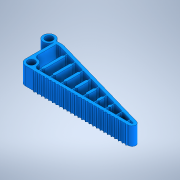
# Autodesk Inventor part: BRAÇO ROBÓTICO - Garra A2
Saved by Autodesk Inventor 2021 (Build 250183000, 183)
## iProperties
Created: 2020-08-23
Part Number: BRAÇO ROBÓTICO - Garra A2
Material: Borracha
Document SubType Name: Modeling
Designer: Araújo, I.
Mass: 6.12763 g
Surface Area: 83.3461 cm^2
Volume: 6.58885 cm^3
Density: 0.93 g/cm^3
Appearance: Borracha - Preta
Author: Araújo, I.
## iProperties of the stored document _3DPrint.ipt
Created: 2020-11-23
Part Number: _3DPrint
Material: Genérico
Document SubType Name: Modeling
Designer: Araújo, I.
Mass: 6.58885 g
Surface Area: 83.3461 cm^2
Volume: 6.58885 cm^3
Density: 1 g/cm^3
Appearance: Padrão
Author: Araújo, I.
Autodesk Inventor part; units mm, degrees
ref_plane "YZ Plane" through (0, 0, 0) normal (1, 0, 0) x (0, 1, 0)
ref_plane "XZ Plane" through (0, 0, 0) normal (0, 1, 0) x (-1, 0, 0)
ref_plane "XY Plane" through (0, 0, 0) normal (0, 0, 1) x (1, 0, 0)
sketch "Esboço1" plane through (0, 0, 0) normal (0, 1, 0) x (-1, 0, 0)
  line L0 (-70.6891, -3.9032) -> (-1.5487, -23.7288)
  arc A0 (-70, 1) -> (-70.6891, -3.9032) centre (-70, -1.5) ccw
  line L1 (-0.9975, -21.8063) -> (-70.1378, -1.9806)
  line L2 (-70, -1) -> (-6, -1)
  line L3 (-7, -20.0851) -> (-7, -18.0851)
  line L4 (-7, -18.0851) -> (-6.4, -17.4851)
  line L5 (-6.4, -17.4851) -> (-6.4, -3.6)
  line L6 (-6.4, -3.6) -> (-7, -3)
  line L7 (-7, -3) -> (-7, -1)
  line L8 (-7.8, -1) -> (-7.8, -3)
  line L9 (-7.8, -3) -> (-8.4, -3.6)
  line L10 (-8.4, -3.6) -> (-8.4, -17.4851)
  line L11 (-8.4, -17.4851) -> (-7.8, -18.0851)
  line L12 (-7.8, -18.0851) -> (-7.8, -19.8557)
  line L13 (-14.5, -17.9345) -> (-14.5, -15.9345)
  line L14 (-14.5, -15.9345) -> (-13.9, -15.3345)
  line L15 (-13.9, -15.3345) -> (-13.9, -3.6)
  line L16 (-13.9, -3.6) -> (-14.5, -3)
  line L17 (-14.5, -3) -> (-14.5, -1)
  line L18 (-15.3, -1) -> (-15.3, -3)
  line L19 (-15.3, -3) -> (-15.9, -3.6)
  line L20 (-15.9, -3.6) -> (-15.9, -15.3345)
  line L21 (-15.9, -15.3345) -> (-15.3, -15.9345)
  line L22 (-15.3, -15.9345) -> (-15.3, -17.7051)
  line L23 (-21.4, -13.1839) -> (-21.4, -3.6)
  line L24 (-23.4, -3.6) -> (-23.4, -13.1839)
  line L25 (-21.4, -3.6) -> (-22, -3)
  line L26 (-22.8, -3) -> (-23.4, -3.6)
  line L27 (-22, -3) -> (-22, -1)
  line L28 (-22.8, -1) -> (-22.8, -3)
  line L29 (-22.8, -13.7839) -> (-22.8, -15.5545)
  line L30 (-23.4, -13.1839) -> (-22.8, -13.7839)
  line L31 (-22, -15.7839) -> (-22, -13.7839)
  line L32 (-22, -13.7839) -> (-21.4, -13.1839)
  line L33 (-28.9, -11.0333) -> (-28.9, -3.6)
  line L34 (-30.9, -3.6) -> (-30.9, -11.0333)
  line L35 (-28.9, -3.6) -> (-29.5, -3)
  line L36 (-30.3, -3) -> (-30.9, -3.6)
  line L37 (-29.5, -3) -> (-29.5, -1)
  line L38 (-30.3, -1) -> (-30.3, -3)
  line L39 (-30.3, -11.6333) -> (-30.3, -13.4039)
  line L40 (-30.9, -11.0333) -> (-30.3, -11.6333)
  line L41 (-29.5, -13.6333) -> (-29.5, -11.6333)
  line L42 (-29.5, -11.6333) -> (-28.9, -11.0333)
  line L43 (-36.4, -8.8827) -> (-36.4, -3.6)
  line L44 (-38.4, -3.6) -> (-38.4, -8.8827)
  line L45 (-36.4, -3.6) -> (-37, -3)
  line L46 (-37.8, -3) -> (-38.4, -3.6)
  line L47 (-37, -3) -> (-37, -1)
  line L48 (-37.8, -1) -> (-37.8, -3)
  line L49 (-37.8, -9.4827) -> (-37.8, -11.2534)
  line L50 (-38.4, -8.8827) -> (-37.8, -9.4827)
  line L51 (-37, -11.4827) -> (-37, -9.4827)
  line L52 (-37, -9.4827) -> (-36.4, -8.8827)
  line L53 (-43.9, -6.7322) -> (-43.9, -3.6)
  line L54 (-45.9, -3.6) -> (-45.9, -6.7322)
  line L55 (-43.9, -3.6) -> (-44.5, -3)
  line L56 (-45.3, -3) -> (-45.9, -3.6)
  line L57 (-44.5, -3) -> (-44.5, -1)
  line L58 (-45.3, -1) -> (-45.3, -3)
  line L59 (-45.3, -7.3322) -> (-45.3, -9.1028)
  line L60 (-45.9, -6.7322) -> (-45.3, -7.3322)
  line L61 (-44.5, -9.3322) -> (-44.5, -7.3322)
  line L62 (-44.5, -7.3322) -> (-43.9, -6.7322)
  line L63 (-51.4, -4.5816) -> (-51.4, -3.6)
  line L64 (-53.4, -3.6) -> (-53.4, -4.5816)
  line L65 (-52, -5.1816) -> (-51.4, -4.5816)
  line L66 (-53.4, -4.5816) -> (-52.8, -5.1816)
  line L67 (-52, -7.1816) -> (-52, -5.1816)
  line L68 (-52.8, -5.1816) -> (-52.8, -6.9522)
  line L69 (-52.8, -3) -> (-53.4, -3.6)
  line L70 (-51.4, -3.6) -> (-52, -3)
  line L71 (-52.8, -1) -> (-52.8, -3)
  line L72 (-52, -3) -> (-52, -1)
  arc A1 (-70, -1) -> (-70.1378, -1.9806) centre (-70, -1.5) ccw
  line L73 (-59.5, -3) -> (-59.5, -1)
  line L74 (-60.3, -1) -> (-60.3, -3)
  line L75 (-58.9, -3.6) -> (-59.5, -3)
  line L76 (-58.9, -2.431) -> (-58.9, -3.6)
  line L77 (-60.3, -3) -> (-60.9, -3.6)
  line L78 (-60.9, -3.6) -> (-60.9, -2.431)
  line L79 (-59.5, -3.031) -> (-58.9, -2.431)
  line L80 (-60.9, -2.431) -> (-60.3, -3.031)
  line L81 (-59.5, -5.031) -> (-59.5, -3.031)
  line L82 (-60.3, -3.031) -> (-60.3, -4.8016)
  line L83 (-67, -2.8804) -> (-67, -1)
  line L84 (-67.8, -2.651) -> (-67.8, -1)
  line L85 (-74.5, -0.7298) -> (-74.5, -1)
  line L86 (-75.3, -0.5004) -> (-75.3, -1)
  circle A2 centre (8, -23) radius 2.5
  arc A3 (4.127, -24) -> (4.127, -22) centre (8, -23) ccw
  line L87 (4.127, -24) -> (0.3807, -24)
  line L88 (4.127, -24) -> (4.127, -22) construction
  arc A4 (-0.9975, -21.8063) -> (0.3807, -22) centre (0.3807, -17) ccw
  arc A5 (-1.5487, -23.7288) -> (0.3807, -24) centre (0.3807, -17) ccw
  circle A6 centre (0, -3) radius 2.5
  line L89 (0, 1) -> (-70, 1)
  arc A7 (-4, -3) -> (-6, -1) centre (-6, -3) ccw
  line L90 (4, -3) -> (4, -22)
  line L91 (2, -9) -> (2, -22)
  arc A8 (-4, -3) -> (0, -7) centre (0, -3) ccw
  arc A9 (4, -3) -> (0, 1) centre (0, -3) ccw
  arc A10 (2, -9) -> (0, -7) centre (0, -9) ccw
  line L92 (4.127, -22) -> (4, -22)
  line L93 (2, -22) -> (0.3807, -22)
  line L94 (-6, -1) -> (-6, 1) construction
  point P0 (4.127, -23)
  point P1 (0, 0)
  point P2 (-6, 0)
  point P3 (-60.3155, -3.0155)
  point P4 (-59.4845, -3.0155)
  dimension "d194" = 16
  dimension "d4" = 2.5
  dimension "d6" = 2
  dimension "d39" = 0.8
  dimension "d40" = 2
  dimension "d41" = 2
  dimension "d44" = 45
  dimension "d46" = 0.8
  dimension "d47" = 2
  dimension "d48" = 2
  dimension "d49" = 45
  dimension "d53" = 7.5
  dimension "d54" = 0.8
  dimension "d55" = 2
  dimension "d56" = 2
  dimension "d57" = 45
  dimension "d63" = 0.8
  dimension "d64" = 2
  dimension "d65" = 2
  dimension "d66" = 45
  dimension "d72" = 0.8
  dimension "d73" = 2
  dimension "d74" = 2
  dimension "d75" = 45
  dimension "d81" = 0.8
  dimension "d82" = 2
  dimension "d83" = 2
  dimension "d84" = 45
  dimension "d117" = 7.5
  dimension "d119" = 7.5
  dimension "d120" = 7.5
  dimension "d124" = 7.5
  dimension "d125" = 0.8
  dimension "d126" = 2
  dimension "d127" = 2
  dimension "d128" = 45
  dimension "d155" = 7.5
  dimension "d157" = 0.8
  dimension "d158" = 2
  dimension "d159" = 2
  dimension "d160" = 45
  dimension "d167" = 7.5
  dimension "d168" = 0.8
  dimension "d169" = 0.8
  dimension "d170" = 7.5
  dimension "d171" = 7.5
  dimension "d183" = 5
  dimension "d184" = 1.5
  dimension "d189" = 5
  dimension "d220" = 5
  dimension "d222" = 70
  dimension "d223" = 20
  dimension "d224" = 8
  dimension "d225" = 7
  dimension "d227" = 2
  dimension "d235" = 2
  dimension "d237" = 1.5
  constraints: 186 end point, 33 point on line, 32 equal length, 21 vertical, 18 horizontal alignment, 18 point on circle, 16 parallel, 13 perpendicular, 11 centre point, 11 tangent, 4 horizontal, 3 coincident, 2 equal radius, 2 midpoint, 1 concentric, 1 vertical alignment, 50 other
  measures "d4" radius of A0
  measures "d39" distance between parallel lines of L8 L7
  measures "d40" distance between parallel lines of L10 L5
  measures "d41" distance of L6.end L7.end
  measures "d44" angle of L11 L12
  measures "d46" distance between parallel lines of L18 L17
  measures "d47" distance between parallel lines of L20 L15
  measures "d48" distance of L16.end L17.end
  measures "d49" angle of L21 L22
  measures "d53" distance between parallel lines of L13 L3
  measures "d54" distance between parallel lines of L28 L27
  measures "d55" distance between parallel lines of L24 L23
  measures "d56" distance of L25.end L27.end
  measures "d57" angle of L30 L29
  measures "d63" distance between parallel lines of L38 L37
  measures "d64" distance between parallel lines of L34 L33
  measures "d65" distance of L35.end L37.end
  measures "d66" angle of L40 L39
  measures "d72" distance between parallel lines of L48 L47
  measures "d73" distance between parallel lines of L44 L43
  measures "d74" distance of L45.end L47.end
  measures "d75" angle of L50 L49
  measures "d81" distance between parallel lines of L58 L57
  measures "d82" distance between parallel lines of L54 L53
  measures "d83" distance of L55.end L57.end
  measures "d84" angle of L60 L59
  measures "d117" distance between parallel lines of L31 L13
  measures "d119" distance between parallel lines of L41 L31
  measures "d120" distance between parallel lines of L51 L41
  measures "d124" distance between parallel lines of L61 L51
  measures "d125" distance between parallel lines of L71 L72
  measures "d126" distance between parallel lines of L64 L63
  measures "d127" distance of L72.start L72.end
  measures "d128" angle of L66 L68
  measures "d155" distance between parallel lines of L67 L61
  measures "d157" distance between parallel lines of L74 L73
  measures "d158" distance between parallel lines of L78 L76
  measures "d159" distance of L73.start L73.end
  measures "d160" angle of L80 L82
  measures "d167" distance between parallel lines of L81 L67
  measures "d168" distance between parallel lines of L84 L83
  measures "d169" distance between parallel lines of L86 L85
  measures "d170" distance between parallel lines of L83 L81
  measures "d171" distance between parallel lines of L85 L83
  measures "d183" diameter of A2
  measures "d184" radial gap between concentric circles of A2 A3
  measures "d189" radius of A4
  measures "d220" diameter of A6
  measures "d222" horizontal distance of A1.centre point (0, 0)
  measures "d223" vertical distance of A6.centre A2.centre
  measures "d224" horizontal distance of A6.centre A2.centre
  measures "d225" distance from line of L3 A6.centre
  measures "d227" radius of A7
  measures "d235" distance between parallel lines of L91 L90
  measures "d237" radial gap between concentric circles of A8 A6
extrude "Extrusão1" add sketch "Esboço1" along normal blind 12 contours A0 L89 A9 L90 L92 A3 L87 A5 L0 | L1 L12 L11 L10 L9 L8 L2 L7 L6 L5 L4 L3 | L1 L22 L21 L20 L19 L18 L2 L17 L16 L15 L14 L13 | L1 L29 L30 L24 L26 L28 L2 L27 L25 L23 L32 L31 | L1 L39 L40 L34 L36 L38 L2 L37 L35 L33 L42 L41 | L1 L49 L50 L44 L46 L48 L2 L47 L45 L43 L52 L51 | L1 L59 L60 L54 L56 L58 L2 L57 L55 L53 L62 L61 | L1 L68 L66 L64 L69 L71 L2 L72 L70 L63 L65 L67 | L1 L82 L80 L77 L74 L2 L73 L75 L79 L81 | L1 L84 L2 L83
sketch "Esboço2" plane through (0, 0, 0) normal (0, 1, 0) x (-1, 0, 0)
  line L0 (-5.8804, 1) -> (-6.3134, 1.75)
  line L1 (-6.4866, 1.75) -> (-6.9196, 1)
  line L2 (-6.9196, 1) -> (-5.8804, 1)
  arc A0 (-6.3134, 1.75) -> (-6.4866, 1.75) centre (-6.4, 1.7) ccw
  line L3 (0, 1) -> (-70, 1) projected
  line L4 (-8.3804, 1) -> (-8.8134, 1.75)
  arc A1 (-8.8134, 1.75) -> (-8.9866, 1.75) centre (-8.9, 1.7) ccw
  line L5 (-8.9866, 1.75) -> (-9.4196, 1)
  line L6 (-9.4196, 1) -> (-8.3804, 1)
  line L7 (-10.8804, 1) -> (-11.3134, 1.75)
  arc A2 (-11.3134, 1.75) -> (-11.4866, 1.75) centre (-11.4, 1.7) ccw
  line L8 (-11.4866, 1.75) -> (-11.9196, 1)
  line L9 (-11.9196, 1) -> (-10.8804, 1)
  line L10 (-13.3804, 1) -> (-13.8134, 1.75)
  arc A3 (-13.8134, 1.75) -> (-13.9866, 1.75) centre (-13.9, 1.7) ccw
  line L11 (-13.9866, 1.75) -> (-14.4196, 1)
  line L12 (-14.4196, 1) -> (-13.3804, 1)
  line L13 (-15.8804, 1) -> (-16.3134, 1.75)
  arc A4 (-16.3134, 1.75) -> (-16.4866, 1.75) centre (-16.4, 1.7) ccw
  line L14 (-16.4866, 1.75) -> (-16.9196, 1)
  line L15 (-16.9196, 1) -> (-15.8804, 1)
  line L16 (-18.3804, 1) -> (-18.8134, 1.75)
  arc A5 (-18.8134, 1.75) -> (-18.9866, 1.75) centre (-18.9, 1.7) ccw
  line L17 (-18.9866, 1.75) -> (-19.4196, 1)
  line L18 (-19.4196, 1) -> (-18.3804, 1)
  line L19 (-20.8804, 1) -> (-21.3134, 1.75)
  arc A6 (-21.3134, 1.75) -> (-21.4866, 1.75) centre (-21.4, 1.7) ccw
  line L20 (-21.4866, 1.75) -> (-21.9196, 1)
  line L21 (-21.9196, 1) -> (-20.8804, 1)
  line L22 (-23.3804, 1) -> (-23.8134, 1.75)
  arc A7 (-23.8134, 1.75) -> (-23.9866, 1.75) centre (-23.9, 1.7) ccw
  line L23 (-23.9866, 1.75) -> (-24.4196, 1)
  line L24 (-24.4196, 1) -> (-23.3804, 1)
  line L25 (-25.8804, 1) -> (-26.3134, 1.75)
  arc A8 (-26.3134, 1.75) -> (-26.4866, 1.75) centre (-26.4, 1.7) ccw
  line L26 (-26.4866, 1.75) -> (-26.9196, 1)
  line L27 (-26.9196, 1) -> (-25.8804, 1)
  line L28 (-28.3804, 1) -> (-28.8134, 1.75)
  arc A9 (-28.8134, 1.75) -> (-28.9866, 1.75) centre (-28.9, 1.7) ccw
  line L29 (-28.9866, 1.75) -> (-29.4196, 1)
  line L30 (-29.4196, 1) -> (-28.3804, 1)
  line L31 (-30.8804, 1) -> (-31.3134, 1.75)
  arc A10 (-31.3134, 1.75) -> (-31.4866, 1.75) centre (-31.4, 1.7) ccw
  line L32 (-31.4866, 1.75) -> (-31.9196, 1)
  line L33 (-31.9196, 1) -> (-30.8804, 1)
  line L34 (-33.3804, 1) -> (-33.8134, 1.75)
  arc A11 (-33.8134, 1.75) -> (-33.9866, 1.75) centre (-33.9, 1.7) ccw
  line L35 (-33.9866, 1.75) -> (-34.4196, 1)
  line L36 (-34.4196, 1) -> (-33.3804, 1)
  line L37 (-35.8804, 1) -> (-36.3134, 1.75)
  arc A12 (-36.3134, 1.75) -> (-36.4866, 1.75) centre (-36.4, 1.7) ccw
  line L38 (-36.4866, 1.75) -> (-36.9196, 1)
  line L39 (-36.9196, 1) -> (-35.8804, 1)
  line L40 (-38.3804, 1) -> (-38.8134, 1.75)
  arc A13 (-38.8134, 1.75) -> (-38.9866, 1.75) centre (-38.9, 1.7) ccw
  line L41 (-38.9866, 1.75) -> (-39.4196, 1)
  line L42 (-39.4196, 1) -> (-38.3804, 1)
  line L43 (-40.8804, 1) -> (-41.3134, 1.75)
  arc A14 (-41.3134, 1.75) -> (-41.4866, 1.75) centre (-41.4, 1.7) ccw
  line L44 (-41.4866, 1.75) -> (-41.9196, 1)
  line L45 (-41.9196, 1) -> (-40.8804, 1)
  line L46 (-43.3804, 1) -> (-43.8134, 1.75)
  arc A15 (-43.8134, 1.75) -> (-43.9866, 1.75) centre (-43.9, 1.7) ccw
  line L47 (-43.9866, 1.75) -> (-44.4196, 1)
  line L48 (-44.4196, 1) -> (-43.3804, 1)
  line L49 (-45.8804, 1) -> (-46.3134, 1.75)
  arc A16 (-46.3134, 1.75) -> (-46.4866, 1.75) centre (-46.4, 1.7) ccw
  line L50 (-46.4866, 1.75) -> (-46.9196, 1)
  line L51 (-46.9196, 1) -> (-45.8804, 1)
  line L52 (-48.3804, 1) -> (-48.8134, 1.75)
  arc A17 (-48.8134, 1.75) -> (-48.9866, 1.75) centre (-48.9, 1.7) ccw
  line L53 (-48.9866, 1.75) -> (-49.4196, 1)
  line L54 (-49.4196, 1) -> (-48.3804, 1)
  line L55 (-50.8804, 1) -> (-51.3134, 1.75)
  arc A18 (-51.3134, 1.75) -> (-51.4866, 1.75) centre (-51.4, 1.7) ccw
  line L56 (-51.4866, 1.75) -> (-51.9196, 1)
  line L57 (-51.9196, 1) -> (-50.8804, 1)
  line L58 (-53.3804, 1) -> (-53.8134, 1.75)
  arc A19 (-53.8134, 1.75) -> (-53.9866, 1.75) centre (-53.9, 1.7) ccw
  line L59 (-53.9866, 1.75) -> (-54.4196, 1)
  line L60 (-54.4196, 1) -> (-53.3804, 1)
  line L61 (-55.8804, 1) -> (-56.3134, 1.75)
  arc A20 (-56.3134, 1.75) -> (-56.4866, 1.75) centre (-56.4, 1.7) ccw
  line L62 (-56.4866, 1.75) -> (-56.9196, 1)
  line L63 (-56.9196, 1) -> (-55.8804, 1)
  line L64 (-58.3804, 1) -> (-58.8134, 1.75)
  arc A21 (-58.8134, 1.75) -> (-58.9866, 1.75) centre (-58.9, 1.7) ccw
  line L65 (-58.9866, 1.75) -> (-59.4196, 1)
  line L66 (-59.4196, 1) -> (-58.3804, 1)
  line L67 (-60.8804, 1) -> (-61.3134, 1.75)
  arc A22 (-61.3134, 1.75) -> (-61.4866, 1.75) centre (-61.4, 1.7) ccw
  line L68 (-61.4866, 1.75) -> (-61.9196, 1)
  line L69 (-61.9196, 1) -> (-60.8804, 1)
  line L70 (-63.3804, 1) -> (-63.8134, 1.75)
  arc A23 (-63.8134, 1.75) -> (-63.9866, 1.75) centre (-63.9, 1.7) ccw
  line L71 (-63.9866, 1.75) -> (-64.4196, 1)
  line L72 (-64.4196, 1) -> (-63.3804, 1)
  line L73 (-65.8804, 1) -> (-66.3134, 1.75)
  arc A24 (-66.3134, 1.75) -> (-66.4866, 1.75) centre (-66.4, 1.7) ccw
  line L74 (-66.4866, 1.75) -> (-66.9196, 1)
  line L75 (-66.9196, 1) -> (-65.8804, 1)
  line L76 (-68.3804, 1) -> (-68.8134, 1.75)
  arc A25 (-68.8134, 1.75) -> (-68.9866, 1.75) centre (-68.9, 1.7) ccw
  line L77 (-68.9866, 1.75) -> (-69.4196, 1)
  line L78 (-69.4196, 1) -> (-68.3804, 1)
  point P0 (0, 0)
  point P1 (-6.4, 1)
  point P2 (-8.9, 1)
  point P3 (-11.4, 1)
  point P4 (-13.9, 1)
  point P5 (-16.4, 1)
  point P6 (-18.9, 1)
  point P7 (-21.4, 1)
  point P8 (-23.9, 1)
  point P9 (-26.4, 1)
  point P10 (-28.9, 1)
  point P11 (-31.4, 1)
  point P12 (-33.9, 1)
  point P13 (-36.4, 1)
  point P14 (-38.9, 1)
  point P15 (-41.4, 1)
  point P16 (-43.9, 1)
  point P17 (-46.4, 1)
  point P18 (-48.9, 1)
  point P19 (-51.4, 1)
  point P20 (-53.9, 1)
  point P21 (-56.4, 1)
  point P22 (-58.9, 1)
  point P23 (-61.4, 1)
  point P24 (-63.9, 1)
  point P25 (-66.4, 1)
  point P26 (-68.9, 1)
  point P27 (-69.4196, 1)
  point P28 (-68.3804, 1)
  point P29 (-66.9196, 1)
  point P30 (-65.8804, 1)
  point P31 (-64.4196, 1)
  point P32 (-63.3804, 1)
  point P33 (-61.9196, 1)
  point P34 (-60.8804, 1)
  point P35 (-59.4196, 1)
  point P36 (-58.3804, 1)
  point P37 (-56.9196, 1)
  point P38 (-55.8804, 1)
  point P39 (-54.4196, 1)
  point P40 (-53.3804, 1)
  point P41 (-51.9196, 1)
  point P42 (-50.8804, 1)
  point P43 (-49.4196, 1)
  point P44 (-48.3804, 1)
  point P45 (-46.9196, 1)
  point P46 (-45.8804, 1)
  point P47 (-39.4196, 1)
  point P48 (-38.3804, 1)
  point P49 (-44.4196, 1)
  point P50 (-43.3804, 1)
  point P51 (-41.9196, 1)
  point P52 (-40.8804, 1)
  point P53 (-29.4196, 1)
  point P54 (-28.3804, 1)
  point P55 (-31.9196, 1)
  point P56 (-30.8804, 1)
  point P57 (-34.4196, 1)
  point P58 (-33.3804, 1)
  point P59 (-36.9196, 1)
  point P60 (-35.8804, 1)
  point P61 (-26.9196, 1)
  point P62 (-25.8804, 1)
  point P63 (-24.4196, 1)
  point P64 (-23.3804, 1)
  point P65 (-21.9196, 1)
  point P66 (-20.8804, 1)
  point P67 (-19.4196, 1)
  point P68 (-18.3804, 1)
  point P69 (-16.9196, 1)
  point P70 (-15.8804, 1)
  point P71 (-14.4196, 1)
  point P72 (-13.3804, 1)
  dimension "d207" = 0.8
  dimension "d208" = 60
  dimension "d209" = 6.4
  dimension "d217" = 0.1
  dimension "d230" = 2.5
  constraints: 156 end point, 150 horizontal alignment, 52 point on circle, 50 parallel, 26 centre point, 25 collinear, 25 equal radius, 2 horizontal, 2 tangent, 1 midpoint, 1 vertical alignment, 1 other
  measures "d208" angle of L0 L2
  measures "d209" horizontal distance of A0.centre point (0, 0)
  measures "d217" radius of A0
  measures "d230" distance of L0.start L4.start
extrude "Extrusão2" add sketch "Esboço2" along normal up to surface (12 mm away)
sketch "Esboço3" plane through (0, 0, 0) normal (0, -1, 0) x (1, 0, 0)
  line L0 (0, 1) -> (5.8804, 1) projected
  arc A0 (0, 1) -> (-4, -3) centre (0, -3) ccw projected
  line L1 (-4, -22) -> (-4, -3) projected
  arc A1 (-4.127, -22) -> (-4.127, -24) centre (-8, -23) ccw projected
  line L2 (-4.127, -22) -> (-4, -22) projected
  line L3 (-0.3807, -24) -> (-4.127, -24) projected
  arc A2 (70.6891, -3.9032) -> (70, 1) centre (70, -1.5) ccw projected
  arc A3 (70.6891, -8.9683) -> (70, 6) centre (70, -1.5) ccw
  line L4 (70, 6) -> (70, 1)
  line L5 (70.6891, -8.9683) -> (70.6891, -3.9032)
  line L6 (-0.3807, -29) -> (-1.2918, -29)
  arc A4 (-9, -14.0557) -> (-1.2918, -29) centre (-8, -23) ccw
  line L7 (-9, -14.0557) -> (-9, -3)
  arc A5 (0, 6) -> (-9, -3) centre (0, -3) ccw
  line L8 (0, 6) -> (0, 1)
  line L9 (-0.3807, -29) -> (-0.3807, -24)
  point P0 (0, 0)
  dimension "d238" = 5
  dimension "d239" = 5
  constraints: 12 end point, 6 point on circle, 4 vertical, 3 centre point, 3 other
  measures "d238" radial gap between concentric circles of A2 A3
  measures "d239" radial gap between concentric circles of A0 A5
equation "\"d47\" = d40"
equation "\"d48\" = d41"
equation "\"d49\" = d44"
equation "\"d57\" = d60"
equation "\"d66\" = d69"
equation "\"d75\" = d78"
equation "\"d84\" = d87"
equation "\"d60\" = 45deg"
equation "\"d69\" = 45deg"
equation "\"d78\" = 45deg"
equation "\"d87\" = 45deg"
